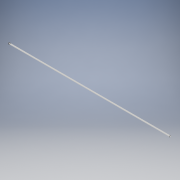
# Autodesk Inventor part: Tc-2
Saved by Autodesk Inventor 2017 (Build 210142000, 142)
## iProperties
Created: 2017-07-13
Part Number: Tc-2
Material: Generic
Document SubType Name: Modeling
Designer: cas7
Density: 1 g/cm^3
Appearance: Default
Author: cas7
Autodesk Inventor part; units mm, degrees
ref_plane "YZ Plane" through (0, 0, 0) normal (1, 0, 0) x (0, 1, 0)
ref_plane "XZ Plane" through (0, 0, 0) normal (0, 1, 0) x (-1, 0, 0)
ref_plane "XY Plane" through (0, 0, 0) normal (0, 0, 1) x (1, 0, 0)
sketch "Sketch1" plane through (0, 0, 0) normal (0, 0, 1) x (1, 0, 0)
  line L0 (0, 1.5875) -> (0, 3.175)
  line L1 (0, 3.175) -> (0, 1.5875)
  line L2 (0, 1.5875) -> (2.5414, 1.5875)
  arc A0 (2.5414, 1.5875) -> (0, 3.175) centre (-0.0802, 0.2187) ccw
  line L3 (0, 1.5875) -> (-230, 1.5875)
  line L4 (-230, 1.5875) -> (-400, 1.5875)
  line L5 (0, 3.175) -> (-400, 3.175)
  line L6 (-400, 3.175) -> (-400, 1.5875)
  line L7 (-400, 3.175) -> (-402.3464, 3.6825)
  line L8 (-402.3393, 1.5875) -> (-402.3464, 3.6825)
  line L9 (-400, 1.5875) -> (-402.3393, 1.5875)
  line L10 (-402.3393, 1.5875) -> (-403.6093, 1.5875)
  line L11 (-403.6093, 1.5875) -> (-403.6093, 3.175)
  line L12 (-403.6093, 3.175) -> (-402.3447, 3.175)
  point P0 (0, 0)
  dimension "d0" = 3.175
  dimension "d5" = 230
  dimension "d6" = 170
  dimension "d7" = 400
  dimension "d9" = 1.27
  dimension "d11" = 1.5875
  constraints: 26 end point, 4 horizontal, 3 point on line, 2 point on circle, 2 vertical, 1 centre point
  measures "d0" distance of point (0, 0) L0.end
  measures "d5" distance of L0.start L3.end
  measures "d6" distance of L3.end L4.end
  measures "d7" distance of L0.end L5.end
  measures "d9" distance of L8.start L10.end
  measures "d11" distance of L10.end L11.end
revolve "Revolution1" add sketch "Sketch1" angle 360 about axis through (-230, 1.5875, 0) along (-1, 0, 0) contours L3 L4 L6 L5 L0 | L0 A0 L2 | L6 L9 L8 L7
revolve "Revolution2" add sketch "Sketch1" angle 360 about axis through (-402.3393, 1.5875, 0) along (-1, 0, 0) contours L10 L11 L12 L8
body "Solid1"
